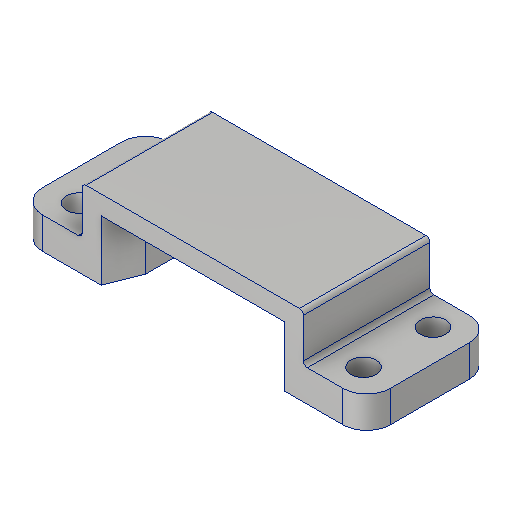
# Autodesk Inventor part: CNCM_ALU_Visial_inspection_tray_bucket_mount
Saved by Autodesk Inventor 2025 (Build 290162010, 162A)
## iProperties
Created: 2018-09-18
Part Number: CNCM_ALU_Visial_inspection_tray_bucket_mount
Material: Aluminum 6061
Document SubType Name: Modeling
Designer: Andrzej
Density: 2.7 g/cm^3
Appearance: Aluminum - Flat
Mass: 1.11888 g
Surface Area: 5.93912 cm^2
Volume: 0.414399 cm^3
Author: Andrzej
Autodesk Inventor part; units mm, degrees
ref_plane "YZ Plane" through (0, 0, 0) normal (1, 0, 0) x (0, 1, 0)
ref_plane "XZ Plane" through (0, 0, 0) normal (0, 1, 0) x (-1, 0, 0)
ref_plane "XY Plane" through (0, 0, 0) normal (0, 0, 1) x (1, 0, 0)
sketch "Sketch1" plane through (0, 0, 0) normal (0, 0, 1) x (1, 0, 0)
  line L0 (-5.7995, -0.4901) -> (0.2005, -0.4901)
  line L1 (0.2005, -0.4901) -> (0.2005, 2.5099)
  line L2 (0.2005, 2.5099) -> (10.2005, 2.5099)
  line L3 (10.2005, 2.5099) -> (10.2005, -0.4901)
  line L4 (10.2005, -0.4901) -> (16.2005, -0.4901)
  line L5 (16.2005, -0.4901) -> (16.2005, 1.5099)
  line L6 (16.2005, 1.5099) -> (12.2005, 1.5099)
  line L7 (12.2005, 1.5099) -> (12.2005, 4.5099)
  line L8 (12.2005, 4.5099) -> (-1.7995, 4.5099)
  line L9 (-1.7995, 4.5099) -> (-1.7995, 1.5099)
  line L10 (-1.7995, 1.5099) -> (-5.7995, 1.5099)
  line L11 (-5.7995, 1.5099) -> (-5.7995, -0.4901)
  point P0 (0, 0)
  dimension "d0" = 3
  dimension "d1" = 2
  dimension "d2" = 2
  dimension "d3" = 2
  dimension "d4" = 2
  dimension "d5" = 2
  dimension "d6" = 10
  dimension "d7" = 6
  dimension "d8" = 6
  constraints: 24 end point, 10 perpendicular, 2 point on line, 1 horizontal
  measures "d0" distance between parallel lines of L2 L0
  measures "d1" distance between parallel lines of L0 L10
  measures "d2" distance between parallel lines of L9 L1
  measures "d3" distance between parallel lines of L2 L8
  measures "d4" distance between parallel lines of L3 L7
  measures "d5" distance between parallel lines of L4 L6
  measures "d6" distance between parallel lines of L3 L1
  measures "d7" distance between parallel lines of L5 L3
  measures "d8" distance of L0.start L0.end
extrude "Extrusion1" add sketch "Sketch1" along normal blind 8
sketch "Sketch2" plane through (12.2005, 1.5099, 0) normal (0, 1, 0) x (1, 0, 0)
  line L0 (-14, 0) -> (-18, 0) projected
  line L1 (-18, 0) -> (-18, -8) projected
  line L2 (-14, -8) -> (-18, -8) projected
  line L3 (-14, 0) -> (-14, -8) projected
  line L4 (4, 0) -> (0, 0) projected
  line L5 (0, 0) -> (0, -8) projected
  line L6 (4, -8) -> (0, -8) projected
  line L7 (4, 0) -> (4, -8) projected
  point P0 (-12.2005, 0)
  point P1 (-16, -1.8)
  point P2 (-16, -6.2)
  point P3 (2, -1.8)
  point P4 (2, -6.2)
  dimension "d11" = 1.8
  dimension "d12" = 1.8
  dimension "d13" = 2
  dimension "d14" = 2
  constraints: 2 horizontal alignment, 2 vertical alignment
  measures "d11" distance from line of L0 point (-16, -1.8)
  measures "d12" distance from line of L2 point (-16, -6.2)
  measures "d13" distance from line of L1 point (-16, -1.8)
  measures "d14" distance from line of L7 point (2, -1.8)
hole "Hole1" at (-3.7995, 1.5099, 1.8) at (-3.7995, 1.5099, 6.2) at (14.2005, 1.5099, 1.8) at (14.2005, 1.5099, 6.2) direction (0, -1, 0) diameter 1.6 depth 8 tip angle 118
fillet "Fillet1" radius 1.5 4 edges at (16.2005, 0.5099, 0) (16.2005, 0.5099, 8) (-5.7995, 0.5099, 0) (-5.7995, 0.5099, 8)
fillet "Fillet2" radius 0.25 4 edges at (12.2005, 4.5099, 4) (12.2005, 1.5099, 4) (-1.7995, 1.5099, 4) (-1.7995, 4.5099, 4)
chamfer "Chamfer1" distance 0.8 distance2 2 1 edges at (5.2005, 2.5099, 8) measured on face at (3.5338, 3.8432, 8)
chamfer "Chamfer2" distance 0.8 distance2 2 1 edges at (0.2005, 1.0099, 8) measured on face at (3.5338, 4.1099, 8)
chamfer "Chamfer3" distance 0.8 distance2 2 1 edges at (10.2005, 1.0099, 8) measured on face at (3.5338, 4.1099, 8)
equation "\"d2\" = d1"
equation "\"d3\" = d1"
equation "\"d4\" = d1"
equation "\"d5\" = d1"
equation "\"d7\" = d8"
equation "\"d12\" = d11"
equation "\"d14\" = d13"
body "Solid1"
